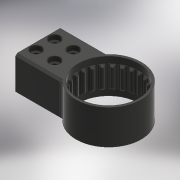
# Autodesk Inventor part: output_housing
Saved by Autodesk Inventor 2020.3 (Build 243373000, 373)
## iProperties
Created: 2021-02-25
Part Number: output_housing
Material: ABS Plastic
Document SubType Name: Modeling
Designer: paulg
Density: 1.06 g/cm^3
Appearance: Smooth - Black
Author: paulg
Autodesk Inventor part; units mm, degrees
ref_plane "YZ Plane" through (0, 0, 0) normal (1, 0, 0) x (0, 1, 0)
ref_plane "XZ Plane" through (0, 0, 0) normal (0, 1, 0) x (-1, 0, 0)
ref_plane "XY Plane" through (0, 0, 0) normal (0, 0, 1) x (1, 0, 0)
sketch "Sketch1" plane through (0, 0, 0) normal (0, 0, 1) x (1, 0, 0)
  line L0 (0, 0) -> (31.65, 0) construction
  circle A0 centre (31.65, 0) radius 1.9
  circle A1 centre (0, 0) radius 32.5 construction
  dimension "d0" = 3.8
  dimension "d1" = 31.65
  dimension "d11" = 65
  constraints: 2 centre point, 2 coincident, 2 end point, 1 horizontal
  measures "d0" diameter of A0
  measures "d1" distance of L0.start L0.end
  measures "d11" diameter of A1
extrude "Extrusion1" add sketch "Sketch1" along normal mid plane 23
pattern_circular "Circular Pattern1" count 25 over 360 about axis through (0, 0, -10) along (0, 0, 1) of "Extrusion1"
sketch "Sketch2" plane through (0, 0, 0) normal (0, 0, 1) x (1, 0, 0)
  circle A0 centre (0, 0) radius 32.6
  circle A1 centre (0, 0) radius 35
  dimension "d7" = 65.2
  dimension "d8" = 70
  constraints: 2 centre point, 2 coincident
  measures "d7" diameter of A0
  measures "d8" diameter of A1
extrude "Extrusion2" add sketch "Sketch2" along normal mid plane 37
fillet "Fillet1" radius 1.5 4 edges at (32.5572, 1.6694, -5.75) (32.5572, 1.6694, 5.75) (32.5572, -1.6694, 5.75) (32.5572, -1.6694, -5.75)
pattern_circular "Circular Pattern2" count 25 over 360 about axis through (0, 0, -10) along (0, 0, 1) of "Fillet1"
sketch "Sketch3" plane through (0, 0, 0) normal (0, 0, 1) x (1, 0, 0)
  circle A0 centre (0, 0) radius 35 projected
  line L0 (0, 0) -> (-49.7474, 0) construction
  line L1 (-75, -25) -> (-24.4949, -25)
  line L2 (-24.4949, -25) -> (-24.4949, 25) construction
  line L3 (-24.4949, 25) -> (-75, 25)
  line L4 (-75, 25) -> (-75, -25)
  line L5 (-75, -25) -> (-24.4949, 25) construction
  line L6 (-24.4949, -25) -> (-75, 25) construction
  arc A1 (-24.4949, 25) -> (-24.4949, -25) centre (0, 0) ccw
  dimension "d16" = 75
  dimension "d17" = 50
  constraints: 14 end point, 2 horizontal, 2 midpoint, 2 parallel, 2 point on circle, 1 centre point, 1 coincident, 1 perpendicular, 2 other
  measures "d16" distance from line of point (0, 0) L4
  measures "d17" distance of L3.end L1.start
extrude "Extrusion3" add sketch "Sketch3" along normal up to surface (37 mm away) from surface at -18.5 contours A0 L1 L4 L3
sketch "Sketch4" plane through (0, 0, 0) normal (0, 1, 0) x (-1, 0, 0)
  line L0 (0, 0) -> (0, -11.5)
  line L1 (0, -11.5) -> (-31.5, -11.5)
  line L2 (-31.5, -11.5) -> (-29.5, -9.5)
  line L3 (-29.5, -9.5) -> (-29.5, -11.5)
  line L4 (-32.6, 18.5) -> (32.6, 18.5) projected
  line L5 (32.6, -18.5) -> (-32.6, -18.5) projected
  line L6 (-26.7271, 11.5) -> (-30.0814, 11.5) projected
  line L7 (-30.0814, -11.5) -> (-26.7271, -11.5) projected
  line L8 (-21.2453, 11.5) -> (-26.0116, 11.5) projected
  line L9 (-26.0116, -11.5) -> (-21.2453, -11.5) projected
  line L10 (-14.4286, 11.5) -> (-20.3075, 11.5) projected
  line L11 (-20.3075, -11.5) -> (-14.4286, -11.5) projected
  line L12 (-6.7054, 11.5) -> (-13.3273, 11.5) projected
  line L13 (-13.3273, -11.5) -> (-6.7054, -11.5) projected
  line L14 (1.4392, 11.5) -> (-5.5098, 11.5) projected
  line L15 (-5.5098, -11.5) -> (1.4392, -11.5) projected
  line L16 (9.4934, 11.5) -> (2.654, 11.5) projected
  line L17 (2.654, -11.5) -> (9.4934, -11.5) projected
  line L18 (16.9511, 11.5) -> (10.651, 11.5) projected
  line L19 (10.651, -11.5) -> (16.9511, -11.5) projected
  line L20 (23.3436, 11.5) -> (17.9788, 11.5) projected
  line L21 (17.9788, -11.5) -> (23.3436, -11.5) projected
  line L22 (28.2694, 11.5) -> (24.1768, 11.5) projected
  line L23 (24.1768, -11.5) -> (28.2694, -11.5) projected
  line L24 (31.419, 11.5) -> (28.8558, 11.5) projected
  line L25 (28.8558, -11.5) -> (31.419, -11.5) projected
  line L26 (32.5943, 11.5) -> (31.7217, 11.5) projected
  line L27 (31.7217, -11.5) -> (32.5943, -11.5) projected
  line L28 (31.7217, 11.5) -> (32.5943, 11.5) projected
  line L29 (32.5943, -11.5) -> (31.7217, -11.5) projected
  line L30 (28.8558, 11.5) -> (31.419, 11.5) projected
  line L31 (31.419, -11.5) -> (28.8558, -11.5) projected
  line L32 (24.1768, 11.5) -> (28.2694, 11.5) projected
  line L33 (28.2694, -11.5) -> (24.1768, -11.5) projected
  line L34 (17.9788, 11.5) -> (23.3436, 11.5) projected
  line L35 (23.3436, -11.5) -> (17.9788, -11.5) projected
  line L36 (10.651, 11.5) -> (16.9511, 11.5) projected
  line L37 (16.9511, -11.5) -> (10.651, -11.5) projected
  line L38 (2.654, 11.5) -> (9.4934, 11.5) projected
  line L39 (9.4934, -11.5) -> (2.654, -11.5) projected
  line L40 (-5.5098, 11.5) -> (1.4392, 11.5) projected
  line L41 (1.4392, -11.5) -> (-5.5098, -11.5) projected
  line L42 (-13.3273, 11.5) -> (-6.7054, 11.5) projected
  line L43 (-6.7054, -11.5) -> (-13.3273, -11.5) projected
  line L44 (-20.3075, 11.5) -> (-14.4286, 11.5) projected
  line L45 (-14.4286, -11.5) -> (-20.3075, -11.5) projected
  line L46 (-26.0116, 11.5) -> (-21.2453, 11.5) projected
  line L47 (-21.2453, -11.5) -> (-26.0116, -11.5) projected
  line L48 (-30.0814, 11.5) -> (-26.7271, 11.5) projected
  line L49 (-26.7271, -11.5) -> (-30.0814, -11.5) projected
  line L50 (-32.261, 11.5) -> (-30.5295, 11.5) projected
  line L51 (-30.5295, -11.5) -> (-32.261, -11.5) projected
  line L52 (-32.4136, 11.5) -> (-32.4136, 11.5) projected
  line L53 (-32.4136, -11.5) -> (-32.4136, 11.5) projected
  line L54 (-32.4136, -11.5) -> (-32.4136, -11.5) projected
  line L55 (-32.4136, 11.5) -> (-32.4136, -11.5) projected
  line L56 (-26.7271, -11.5) -> (-26.7271, 11.5) projected
  line L57 (-30.0814, 11.5) -> (-30.0814, -11.5) projected
  line L58 (-21.2453, -11.5) -> (-21.2453, 11.5) projected
  line L59 (-26.0116, 11.5) -> (-26.0116, -11.5) projected
  line L60 (-14.4286, -11.5) -> (-14.4286, 11.5) projected
  line L61 (-20.3075, 11.5) -> (-20.3075, -11.5) projected
  line L62 (-6.7054, -11.5) -> (-6.7054, 11.5) projected
  line L63 (-13.3273, 11.5) -> (-13.3273, -11.5) projected
  line L64 (1.4392, -11.5) -> (1.4392, 11.5) projected
  line L65 (-5.5098, 11.5) -> (-5.5098, -11.5) projected
  line L66 (9.4934, -11.5) -> (9.4934, 11.5) projected
  line L67 (2.654, 11.5) -> (2.654, -11.5) projected
  line L68 (16.9511, -11.5) -> (16.9511, 11.5) projected
  line L69 (10.651, 11.5) -> (10.651, -11.5) projected
  line L70 (23.3436, -11.5) -> (23.3436, 11.5) projected
  line L71 (17.9788, 11.5) -> (17.9788, -11.5) projected
  line L72 (28.2694, -11.5) -> (28.2694, 11.5) projected
  line L73 (24.1768, 11.5) -> (24.1768, -11.5) projected
  line L74 (31.419, -11.5) -> (31.419, 11.5) projected
  line L75 (28.8558, 11.5) -> (28.8558, -11.5) projected
  line L76 (32.5943, -11.5) -> (32.5943, 11.5) projected
  line L77 (31.7217, 11.5) -> (31.7217, -11.5) projected
  line L78 (31.7217, -11.5) -> (31.7217, 11.5) projected
  line L79 (32.5943, 11.5) -> (32.5943, -11.5) projected
  line L80 (28.8558, -11.5) -> (28.8558, 11.5) projected
  line L81 (31.419, 11.5) -> (31.419, -11.5) projected
  line L82 (24.1768, -11.5) -> (24.1768, 11.5) projected
  line L83 (28.2694, 11.5) -> (28.2694, -11.5) projected
  line L84 (17.9788, -11.5) -> (17.9788, 11.5) projected
  line L85 (23.3436, 11.5) -> (23.3436, -11.5) projected
  line L86 (10.651, -11.5) -> (10.651, 11.5) projected
  line L87 (16.9511, 11.5) -> (16.9511, -11.5) projected
  line L88 (2.654, -11.5) -> (2.654, 11.5) projected
  line L89 (9.4934, 11.5) -> (9.4934, -11.5) projected
  line L90 (-5.5098, -11.5) -> (-5.5098, 11.5) projected
  line L91 (1.4392, 11.5) -> (1.4392, -11.5) projected
  line L92 (-13.3273, -11.5) -> (-13.3273, 11.5) projected
  line L93 (-6.7054, 11.5) -> (-6.7054, -11.5) projected
  line L94 (-20.3075, -11.5) -> (-20.3075, 11.5) projected
  line L95 (-14.4286, 11.5) -> (-14.4286, -11.5) projected
  line L96 (-26.0116, -11.5) -> (-26.0116, 11.5) projected
  line L97 (-21.2453, 11.5) -> (-21.2453, -11.5) projected
  line L98 (-30.0814, -11.5) -> (-30.0814, 11.5) projected
  line L99 (-26.7271, 11.5) -> (-26.7271, -11.5) projected
  line L100 (-32.261, -11.5) -> (-32.261, 11.5) projected
  line L101 (-30.5295, 11.5) -> (-30.5295, -11.5) projected
  dimension "d20" = 31.5
  dimension "d21" = 2
  dimension "d22" = 45
  constraints: 8 end point, 1 collinear, 1 parallel, 1 perpendicular, 1 point on line, 1 vertical
  measures "d20" distance of L0.end L1.end
  measures "d21" distance of L2.end L3.end
  measures "d22" angle of L2 L3
revolve "Revolution1" cut sketch "Sketch4" angle 360 about axis through (0, 0, 0) along (0, 0, -1) contours L1 L57 L2 L3 | L1 L101 L2 L57 | L1 L2 L101
mirror "Mirror1" about plane through (0, 0, 0) normal (0, 0, 1) of "Revolution1"
sketch "Sketch5" plane through (-75, -25, 18.5) normal (-1, 0, 0) x (0, 0, 1)
  line L0 (-29, 4.5) -> (-8, 4.5)
  line L1 (-8, 4.5) -> (-8, 45.5)
  line L2 (-8, 45.5) -> (-29, 45.5)
  line L3 (-29, 45.5) -> (-29, 4.5)
  line L4 (-29, 4.5) -> (-8, 45.5) construction
  line L5 (-8, 4.5) -> (-29, 45.5) construction
  line L6 (-29, 44.7929) -> (-28.2929, 45.5)
  line L7 (-28.2929, 45.5) -> (-29, 46.2071)
  line L8 (-29, 46.2071) -> (-29.7071, 45.5)
  line L9 (-29.7071, 45.5) -> (-29, 44.7929)
  line L10 (-29, 44.7929) -> (-29, 46.2071) construction
  line L11 (-28.2929, 45.5) -> (-29.7071, 45.5) construction
  line L12 (-8, 44.7929) -> (-8.7071, 45.5)
  line L13 (-8.7071, 45.5) -> (-8, 46.2071)
  line L14 (-8, 46.2071) -> (-7.2929, 45.5)
  line L15 (-7.2929, 45.5) -> (-8, 44.7929)
  line L16 (-8, 44.7929) -> (-8, 46.2071) construction
  line L17 (-8.7071, 45.5) -> (-7.2929, 45.5) construction
  line L18 (-28.2929, 4.5) -> (-29, 3.7929)
  line L19 (-29, 3.7929) -> (-29.7071, 4.5)
  line L20 (-29.7071, 4.5) -> (-29, 5.2071)
  line L21 (-29, 5.2071) -> (-28.2929, 4.5)
  line L22 (-28.2929, 4.5) -> (-29.7071, 4.5) construction
  line L23 (-29, 3.7929) -> (-29, 5.2071) construction
  line L24 (-8.7071, 4.5) -> (-8, 3.7929)
  line L25 (-8, 3.7929) -> (-7.2929, 4.5)
  line L26 (-7.2929, 4.5) -> (-8, 5.2071)
  line L27 (-8, 5.2071) -> (-8.7071, 4.5)
  line L28 (-8.7071, 4.5) -> (-7.2929, 4.5) construction
  line L29 (-8, 3.7929) -> (-8, 5.2071) construction
  point P0 (-18.5, 25)
  dimension "d24" = 41
  dimension "d25" = 21
  dimension "d26" = 1
  constraints: 60 end point, 11 parallel, 10 midpoint, 6 equal length, 6 perpendicular, 4 horizontal
  measures "d24" distance of L0.end L1.end
  measures "d25" distance of L0.start L0.end
  measures "d26" distance of L7.end L8.end
extrude "Extrusion4" cut sketch "Sketch5" against normal blind 37
chamfer "Chamfer1" distance 2 angle 45 4 edges at (-49.7474, -25, -18.5) (-49.7474, 25, -18.5) (-49.7474, -25, 18.5) (-49.7474, 25, 18.5)
fillet "Fillet2" radius 10 2 edges at (-24.4949, -25, 0) (-24.4949, 25, 0)
sketch "Sketch9" plane through (0, 0, 18.5) normal (0, 0, 1) x (1, 0, 0)
  line L0 (0, 0) -> (-38, 0)
  dimension "d63" = 38
  constraints: 2 end point, 1 horizontal
  measures "d63" distance of L0.start L0.end
sketch "Sketch11" plane through (0, 0, 18.5) normal (0, 0, 1) x (1, 0, 0)
  line L0 (-75, -23) -> (-75, 23) projected
  line L1 (-75, 0) -> (-58, 0)
  line L2 (-68, 10) -> (-48, 10)
  line L3 (-48, 10) -> (-48, -10)
  line L4 (-48, -10) -> (-68, -10)
  line L5 (-68, -10) -> (-68, 10)
  line L6 (-68, 10) -> (-48, -10) construction
  line L7 (-48, 10) -> (-68, -10) construction
  point P0 (0, 0)
  dimension "d67" = 17
  dimension "d68" = 20
  dimension "d69" = 20
  constraints: 14 end point, 3 midpoint, 2 horizontal, 2 parallel, 1 perpendicular
  measures "d67" distance of L1.start L1.end
  measures "d68" distance of L3.end L4.end
  measures "d69" distance of L2.end L3.end
hole "Hole3" at (-68, 10, 18.5) at (-48, 10, 18.5) at (-48, -10, 18.5) at (-68, -10, 18.5) direction (0, 0, -1) diameter 5.5 depth 8 tip angle 118 counterbore diameter 12 counterbore depth 5
mirror "Mirror3" about plane through (0, 0, 0) normal (0, 0, 1) of "Hole3"
equation "\"E_\" = 1"
equation "\"Rr_\" = 2"
equation "\"R_\" = 31.5"
body "Solid1"
